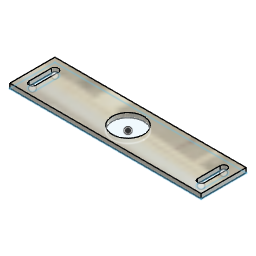
Chumaceira (Autodesk Fusion 360 design; units mm, degrees)
Autodesk Fusion 360 part; units mm, degrees
sketch "Sketch1" plane through (0, 0, 0) normal (0, 1, 0) x (1, 0, 0)
  line L0 (85, -20) -> (-85, -20)
  line L1 (-85, -20) -> (-85, 20)
  line L2 (-85, 20) -> (85, 20)
  line L3 (85, 20) -> (85, -20)
  circle A0 centre (0, 0) radius 14
  line L4 (71.9, 10) -> (71.9, -10)
  arc A1 (71.9, -10) -> (78.1, -10) centre (75, -10) ccw
  line L5 (78.1, -10) -> (78.1, 10)
  arc A2 (78.1, 10) -> (71.9, 10) centre (75, 10) ccw
  line L6 (-71.9, 10) -> (-71.9, -10)
  arc A3 (-71.9, 10) -> (-78.1, 10) centre (-75, 10) ccw
  line L7 (-78.1, -10) -> (-78.1, 10)
  arc A4 (-78.1, -10) -> (-71.9, -10) centre (-75, -10) ccw
  dimension "d1" = 170
  dimension "d2" = 40
  dimension "d4" = 28
  dimension "d7" = 20
  dimension "d10" = 6.2
  dimension "d11" = 150
  constraint horizontal L0
  constraint perpendicular L0 L1
  constraint parallel L0 L2
  constraint parallel L1 L3
  constraint coincident A0.centre origin
  constraint tangent L4 A1
  constraint tangent A1 L5
  constraint parallel L4 L5
  constraint tangent L5 A2
  constraint tangent L4 A2
  measures "d1" distance of L1.end L2.end
  measures "d2" distance of L0.end L1.end
  measures "d4" diameter of A0
  measures "d7" distance of A2.centre A1.centre
  measures "d10" diameter of A1
  measures "d11" distance of A1.centre A4.centre
extrude "Extrude1" add sketch "Sketch1" along normal blind 4
